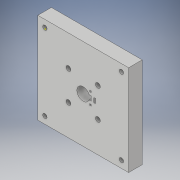
# Autodesk Inventor part: armmount
Saved by Autodesk Inventor 2018 (Build 220112000, 112)
## iProperties
Created: 2017-11-17
Part Number: armmount
Material: Generic
Document SubType Name: Modeling
Designer: 10283
Density: 1 g/cm^3
Appearance: Default
Author: 10283
## iProperties of the stored document armmount_3DPrint.ipt
Created: 2018-06-07
Part Number: armmount_3DPrint
Material: Generic
Document SubType Name: Modeling
Designer: 4070609
Density: 1 g/cm^3
Appearance: Default
Author: 4070609
Autodesk Inventor part; units mm, degrees
ref_plane "YZ Plane" through (0, 0, 0) normal (1, 0, 0) x (0, 1, 0)
ref_plane "XZ Plane" through (0, 0, 0) normal (0, 1, 0) x (-1, 0, 0)
ref_plane "XY Plane" through (0, 0, 0) normal (0, 0, 1) x (1, 0, 0)
sketch "Sketch1" plane through (0, 0, 0) normal (0, 0, 1) x (1, 0, 0)
  line L0 (-6.3269, 6.7325) -> (69.8731, 6.7325)
  line L1 (69.8731, 6.7325) -> (69.8731, -69.4675)
  line L2 (69.8731, -69.4675) -> (-6.3269, -69.4675)
  line L3 (-6.3269, -69.4675) -> (-6.3269, 6.7325)
  line L4 (-6.3269, 6.7325) -> (69.8731, -69.4675) construction
  line L5 (69.8731, 6.7325) -> (-6.3269, -69.4675) construction
  circle A0 centre (31.7731, -31.3675) radius 4.7625
  circle A1 centre (63.9041, 0.7635) radius 1.8161
  circle A2 centre (63.9041, -63.4985) radius 1.8161
  circle A3 centre (-0.3579, -63.4985) radius 1.8161
  circle A4 centre (-0.3579, 0.7635) radius 1.8161
  line L6 (12.7231, -50.4175) -> (50.8231, -50.4175) construction
  line L7 (50.8231, -50.4175) -> (50.8231, -12.3175) construction
  line L8 (50.8231, -12.3175) -> (12.7231, -12.3175) construction
  line L9 (12.7231, -12.3175) -> (12.7231, -50.4175) construction
  line L10 (12.7231, -50.4175) -> (50.8231, -12.3175) construction
  line L11 (50.8231, -50.4175) -> (12.7231, -12.3175) construction
  circle A5 centre (19.416, -19.0104) radius 2.0193
  circle A6 centre (44.1302, -19.0104) radius 2.0193
  circle A7 centre (19.416, -43.7246) radius 2.0193
  circle A8 centre (44.1302, -43.7246) radius 2.0193
  dimension "d0" = 76.2
  dimension "d1" = 76.2
  dimension "d2" = 9.525
  dimension "d4" = 3.6322
  dimension "d5" = 3.6322
  dimension "d6" = 3.6322
  dimension "d7" = 3.6322
  dimension "d11" = 38.1
  dimension "d12" = 38.1
  dimension "d13" = 4.0386
  dimension "d14" = 4.0386
  dimension "d15" = 4.0386
  dimension "d16" = 4.0386
  dimension "d17" = 24.7142
  dimension "d18" = 64.262
  constraints: 24 end point, 9 centre point, 8 point on line, 4 parallel, 4 vertical alignment, 3 horizontal alignment, 3 midpoint, 2 horizontal, 2 perpendicular, 1 coincident
  measures "d0" distance of L1.end L2.end
  measures "d1" distance of L0.end L1.end
  measures "d2" diameter of A0
  measures "d4" diameter of A1
  measures "d5" diameter of A2
  measures "d6" diameter of A3
  measures "d7" diameter of A4
  measures "d11" distance of L8.end L7.end
  measures "d12" distance of L6.end L7.end
  measures "d13" diameter of A5
  measures "d14" diameter of A6
  measures "d15" diameter of A7
  measures "d16" diameter of A8
  measures "d17" distance of A6.centre A5.centre
  measures "d18" distance of A1.centre A4.centre
extrude "Extrusion1" add sketch "Sketch1" along normal blind 11.43
sketch "Sketch2" plane through (0, 0, 11.43) normal (0, 0, 1) x (1, 0, 0)
  circle A0 centre (31.7731, -31.3675) radius 4.7625 construction
  line L0 (27.0106, -31.3675) -> (38.4406, -31.3675) construction
  line L1 (38.4406, -31.3675) -> (38.4406, -29.5895) construction
  line L2 (38.4406, -29.5895) -> (34.9614, -29.5895)
  line L3 (34.9614, -29.5895) -> (34.9614, -33.8756)
  line L4 (34.9614, -33.8756) -> (38.4406, -33.8756)
  line L5 (38.4406, -33.8756) -> (38.4406, -29.5895)
  point P0 (0, 0)
  dimension "d21" = 11.43
  dimension "d22" = 1.778
  constraints: 12 end point, 2 horizontal, 2 parallel, 2 perpendicular, 1 horizontal alignment, 1 other
  measures "d21" distance of L0.start L0.end
  measures "d22" distance of L0.end L1.end
extrude "Extrusion2" cut sketch "Sketch2" along normal through all both and the other way through all
sketch "Sketch3" plane through (0, 0, 11.43) normal (0, 0, 1) x (1, 0, 0)
  line L0 (38.4406, -33.8756) -> (35.8216, -33.8756) projected
  line L1 (38.4406, -29.5895) -> (35.8216, -29.5895)
  line L2 (35.8216, -33.8756) -> (38.4406, -33.8756)
  line L3 (38.4406, -33.8756) -> (38.4406, -29.5895)
  arc A0 (35.8216, -33.8756) -> (36.1912, -29.5895) centre (31.7731, -31.3675) ccw
  line L4 (35.8216, -33.8756) -> (38.4406, -33.8756)
  line L5 (38.4406, -29.5895) -> (36.1912, -29.5895) projected
  line L6 (38.4406, -29.5895) -> (36.1912, -29.5895)
  point P0 (0, 0)
  point P1 (31.7731, -31.3675)
  constraints: 10 end point, 3 equal length, 2 point on circle, 1 centre point, 1 horizontal
extrude "Extrusion3" add sketch "Sketch3" against normal up to surface (11.43 mm away)
sketch "Sketch4" plane through (0, 0, 11.43) normal (0, 0, 1) x (1, 0, 0)
  circle A0 centre (31.7731, -31.3675) radius 4.7625 construction
  line L0 (27.0106, -31.3675) -> (38.4406, -31.3675) construction
  line L1 (38.4406, -31.3675) -> (38.4406, -29.4625) construction
  line L2 (38.4406, -29.4625) -> (38.4406, -33.2725)
  line L3 (38.4406, -33.2725) -> (36.138, -33.2725)
  line L4 (38.4406, -29.4625) -> (36.138, -29.4625)
  arc A1 (36.138, -33.2725) -> (36.138, -29.4625) centre (31.7731, -31.3675) ccw
  point P0 (0, 0)
  dimension "d27" = 11.43
  dimension "d28" = 1.905
  dimension "d29" = 3.81
  constraints: 10 end point, 5 point on circle, 2 parallel, 1 centre point, 1 horizontal, 1 perpendicular, 1 point on line
  measures "d27" distance of L0.start L0.end
  measures "d28" distance of L0.end L1.end
  measures "d29" distance of L1.end L2.end
extrude "Extrusion4" cut sketch "Sketch4" against normal up to surface (11.43 mm away)
sketch "Sketch5" plane through (0, 0, 11.43) normal (0, 0, 1) x (1, 0, 0)
  line L0 (38.4406, -33.2725) -> (38.4406, -29.4625) construction
  line L1 (38.4406, -29.4625) -> (38.4406, -27.0625) construction
  line L2 (38.4406, -33.2725) -> (38.4406, -35.6725) construction
  line L3 (38.4406, -35.6725) -> (37.2928, -35.6725)
  line L4 (37.2928, -35.6725) -> (37.2928, -36.8725)
  line L5 (37.2928, -36.8725) -> (38.4406, -36.8725)
  line L6 (38.4406, -36.8725) -> (38.4406, -35.6725)
  line L7 (38.4406, -27.0625) -> (37.2928, -27.0625)
  line L8 (37.2928, -27.0625) -> (37.2928, -25.8625)
  line L9 (37.2928, -25.8625) -> (38.4406, -25.8625)
  line L10 (38.4406, -25.8625) -> (38.4406, -27.0625)
  arc A0 (36.138, -29.4625) -> (36.138, -33.2725) centre (31.7731, -31.3675) ccw projected
  line L11 (36.138, -29.4625) -> (38.4406, -29.4625) construction
  line L12 (38.4406, -29.4625) -> (40.8406, -29.4625) construction
  line L13 (40.8406, -29.4625) -> (42.0406, -29.4625)
  line L14 (42.0406, -29.4625) -> (42.0406, -33.2725)
  line L15 (42.0406, -33.2725) -> (40.8406, -33.2725)
  line L16 (40.8406, -33.2725) -> (40.8406, -29.4625)
  point P0 (0, 0)
  dimension "d32" = 2.4
  dimension "d33" = 2.4
  dimension "d34" = 1.2
  dimension "d35" = 1.2
  dimension "d36" = 7
  dimension "d37" = 2.4
  dimension "d38" = 1.2
  constraints: 30 end point, 6 parallel, 4 horizontal, 3 perpendicular, 2 vertical, 1 point on line
  measures "d32" distance of L0.end L1.end
  measures "d33" distance of L0.start L2.end
  measures "d34" distance between parallel lines of L7 L9
  measures "d35" distance between parallel lines of L5 L3
  measures "d36" distance of A0.centre L3.end
  measures "d37" distance of L0.end L12.end
  measures "d38" distance of L14.end L15.end
extrude "Extrusion5" cut sketch "Sketch5" against normal blind 25.4
sketch "Sketch6" plane through (0, 0, 11.43) normal (0, 0, 1) x (1, 0, 0)
  point P0 (0, 0)
sketch "Sketch7" plane through (0, 0, 11.43) normal (0, 0, 1) x (1, 0, 0)
  arc A0 (36.138, -29.4625) -> (36.138, -33.2725) centre (31.7731, -31.3675) ccw projected
  circle A1 centre (31.7731, -31.3675) radius 5.3
  point P0 (0, 0)
  dimension "d41" = 10.6
  constraints: 1 centre point, 1 coincident
  measures "d41" diameter of A1
extrude "Extrusion6" cut sketch "Sketch7" against normal through all
body "Solid1"
